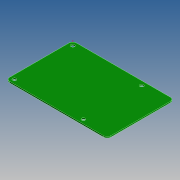
# Autodesk Inventor part: R000
Saved by Autodesk Inventor 2017 (Build 210142000, 142)
## iProperties
Created: 2018-10-05
Part Number: R000
Material: Générique
Document SubType Name: Modeling
Designer: Gilles Mottiez
Density: 1 g/cm^3
Appearance: Vert foncé
Description: Plaque de base Raspberry pi 3B
Author: Gilles Mottiez
Autodesk Inventor part; units mm, degrees
ref_plane "YZ Plane" through (0, 0, 0) normal (1, 0, 0) x (0, 1, 0)
ref_plane "XZ Plane" through (0, 0, 0) normal (0, 1, 0) x (-1, 0, 0)
ref_plane "XY Plane" through (0, 0, 0) normal (0, 0, 1) x (1, 0, 0)
sketch "Sketch1" plane through (0, 0, 0) normal (0, 0, 1) x (1, 0, 0)
  line L0 (0, 0) -> (85, 0)
  line L1 (85, 0) -> (85, -56)
  line L2 (85, -56) -> (0, -56)
  line L3 (0, -56) -> (0, 0)
  dimension "d0" = 85
  dimension "d1" = 56
  constraints: 8 end point, 2 parallel, 1 horizontal, 1 perpendicular
  measures "d0" distance of L1.end L2.end
  measures "d1" distance of L0.end L1.end
extrude "Extrusion1" add sketch "Sketch1" along normal blind 1
fillet "Congé1" radius 3 4 edges at (0, 0, 0.5) (85, 0, 0.5) (85, -56, 0.5) (0, -56, 0.5)
sketch "Esquisse2" plane through (0, 0, 1) normal (0, 0, 1) x (1, 0, 0)
  point P0 (0, 0)
sketch "Esquisse3" plane through (0, 0, 1) normal (0, 0, 1) x (1, 0, 0)
  arc A0 (0, -53) -> (3, -56) centre (3, -53) ccw construction
  line L0 (3, -56) -> (82, -56) construction
  arc A1 (82, -56) -> (85, -53) centre (82, -53) ccw construction
  line L1 (85, -53) -> (85, -3) construction
  arc A2 (85, -3) -> (82, 0) centre (82, -3) ccw construction
  line L2 (82, 0) -> (3, 0) construction
  arc A3 (3, 0) -> (0, -3) centre (3, -3) ccw construction
  line L3 (0, -3) -> (0, -53) construction
  line L4 (3.5, -3.5) -> (61.5, -3.5) construction
  line L5 (61.5, -3.5) -> (61.5, -52.5) construction
  line L6 (61.5, -52.5) -> (3.5, -52.5) construction
  line L7 (3.5, -52.5) -> (3.5, -3.5) construction
  point P0 (0, 0)
  dimension "d5" = 3.5
  dimension "d6" = 49
  dimension "d7" = 58
  dimension "d8" = 3.5
  constraints: 8 end point, 4 coincident, 2 parallel, 1 horizontal, 1 perpendicular
  measures "d5" distance between parallel lines of L0 L6
  measures "d6" distance of L6.end L4.start
  measures "d7" distance of L4.start L4.end
  measures "d8" distance between parallel lines of L3 L7
hole "Perçage1" at (61.5, -52.5, 1) at (3.5, -52.5, 1) at (3.5, -3.5, 1) at (61.5, -3.5, 1) direction (0, 0, -1) diameter 3 end through all
